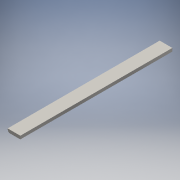
# Autodesk Inventor part: Hydraulic VaneCJE
Saved by Autodesk Inventor 2018 (Build 220112000, 112)
## iProperties
Created: 2018-02-17
Part Number: Hydraulic VaneCJE
Material: Titanium
Document SubType Name: Modeling
Designer: textboox5
Density: 4.51 g/cm^3
Appearance: Titanium
Author: textboox5
Autodesk Inventor part; units mm, degrees
ref_plane "YZ Plane" through (0, 0, 0) normal (1, 0, 0) x (0, 1, 0)
ref_plane "XZ Plane" through (0, 0, 0) normal (0, 1, 0) x (-1, 0, 0)
sketch "Sketch1" plane through (0, 0, 0) normal (0, 0, 1) x (1, 0, 0)
  line L0 (-152.4, -12.7) -> (-253.6823, -12.7) construction
  line L1 (-152.4, 12.7) -> (-152.4, -12.7) construction
  line L2 (-253.6823, 12.7) -> (-152.4, 12.7) construction
  line L3 (-165.1, -12.7) -> (-165.1, 12.7)
  line L4 (-165.1, 12.7) -> (-266.7, 12.7)
  arc A0 (-266.7, 12.7) -> (-261.5956, -6.35) centre (-228.6, 12.7) ccw
  line L5 (-165.1, -12.7) -> (-250.597, -12.7)
  arc A1 (-261.5956, -6.35) -> (-250.597, -12.7) centre (-250.597, 0) ccw
  point P0 (0, 0)
  point P1 (-256.9981, -12.7)
  dimension "d0" = 38.1
  dimension "d1" = 12.7
  dimension "d4" = 101.6
  constraints: 6 end point, 5 point on circle, 4 point on line, 2 centre point, 2 perpendicular, 2 tangent, 1 horizontal
  measures "d0" distance of L4.end A0.centre
  measures "d1" radius of A1
  measures "d4" distance of L3.end L4.end
ref_plane "Work Plane1" through (-253.6823, -254, -1219.2) normal (0, 0, -1) x (0, 1, 0)
extrude "Extrusion1" add sketch "Sketch1" against normal up to surface (1219.2 mm away)
body "Solid1"
